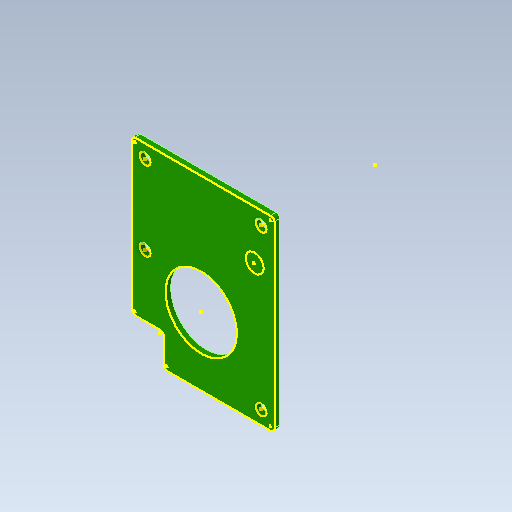
# Autodesk Inventor part: LED_PCB
Saved by Autodesk Inventor 2021 (Build 250183000, 183)
## iProperties
Created: 2020-02-27
Part Number: LED_PCB
Material: Generic
Document SubType Name: Modeling
Designer: lgnds
Density: 1 g/cm^3
Appearance: Default
Author: lgnds
Autodesk Inventor part; units mm, degrees
ref_plane "YZ Plane" through (0, 0, 0) normal (1, 0, 0) x (0, 1, 0)
ref_plane "XZ Plane" through (0, 0, 0) normal (0, 1, 0) x (-1, 0, 0)
ref_plane "XY Plane" through (0, 0, 0) normal (0, 0, 1) x (1, 0, 0)
sketch "Sketch1" plane through (0, 0, 0) normal (0, 0, 1) x (1, 0, 0)
  line L0 (-69, -79.6965) -> (69, -79.6965)
  line L1 (69, -79.6965) -> (69, 79.6965)
  line L2 (69, 79.6965) -> (-69, 79.6965)
  line L3 (-69, 79.6965) -> (-69, -79.6965)
  line L4 (-69, -79.6965) -> (69, 79.6965) construction
  line L5 (69, -79.6965) -> (-69, 79.6965) construction
  point P0 (0, 0)
  dimension "d0" = 138
  dimension "d1" = 159.393
  constraints: 12 end point, 2 midpoint, 2 parallel, 1 horizontal, 1 perpendicular
  measures "d0" distance of L1.end L2.end
  measures "d1" distance of L2.end L0.start
extrude "Extrusion1" add sketch "Sketch1" along normal blind 1.6
sketch "Sketch2" plane through (0, 0, 1.6) normal (0, 0, 1) x (1, 0, 0)
  line L0 (-69, -79.6965) -> (69, -79.6965) projected
  line L1 (69, -79.6965) -> (-23, -79.6965)
  line L2 (-23, -79.6965) -> (-23, -26.0895)
  line L3 (-23, -26.0895) -> (69, -26.0895)
  line L4 (69, -26.0895) -> (69, -79.6965)
  point P0 (0, 0)
  dimension "d4" = 53.607
  dimension "d5" = 92
  constraints: 8 end point, 2 parallel, 1 horizontal, 1 perpendicular
  measures "d4" distance between parallel lines of L3 L0
  measures "d5" distance of L2.end L3.end
extrude "Extrusion2" cut sketch "Sketch2" against normal blind 1.6
sketch "Sketch3" plane through (0, 0, 1.6) normal (0, 0, 1) x (1, 0, 0)
  line L0 (-86.2964, 75.1965) -> (76.951, 75.1965) construction
  line L1 (69, 79.6965) -> (-69, 79.6965) projected
  circle A0 centre (-42, 75.1965) radius 1.6
  circle A1 centre (42, 75.1965) radius 1.6
  line L2 (-69, 79.6965) -> (-69, -79.6965) projected
  line L3 (69, -26.0895) -> (69, 79.6965) projected
  point P0 (0, 0)
  dimension "d8" = 4.5
  dimension "d9" = 27
  dimension "d10" = 27
  dimension "d11" = 3.2
  dimension "d12" = 3.2
  constraints: 2 centre point, 2 end point, 2 point on line, 1 horizontal
  measures "d8" distance between parallel lines of L1 L0
  measures "d9" distance from line of L2 A0.centre
  measures "d10" distance from line of L3 A1.centre
  measures "d11" diameter of A0
  measures "d12" diameter of A1
extrude "Extrusion3" cut sketch "Sketch3" against normal blind 1.6
sketch "Sketch4" plane through (0, 0, 1.6) normal (0, 0, 1) x (1, 0, 0)
  circle A0 centre (-64.5, 12.6965) radius 2 construction
  circle A1 centre (-64.5, 62.6965) radius 2 construction
  circle A2 centre (0, 75.1965) radius 1.5 construction
  circle A3 centre (64.5, 52.6965) radius 1.5 construction
  circle A4 centre (64.5, 23) radius 1.5 construction
  circle A5 centre (64.5, -21.1966) radius 1.5 construction
  circle A6 centre (42, -21.1966) radius 1.5 construction
  circle A7 centre (0, -21.1966) radius 1.5 construction
  circle A8 centre (-32, -30.1966) radius 1.5 construction
  circle A9 centre (-32, -75.1966) radius 1.5 construction
  circle A10 centre (-64.5, -52.6966) radius 1.5 construction
  circle A11 centre (-64.5, -30.1966) radius 1.5 construction
  circle A12 centre (-64.5, 23) radius 1.5 construction
  circle A13 centre (-64.5, 52.6965) radius 1.5 construction
  circle A14 centre (-48.8035, -60) radius 7.75 construction
  arc A15 (-64.5, 57.6965) -> (-64.5, 67.6965) centre (-64.5, 62.6965) ccw
  line L0 (-64.5, 67.6965) -> (-69, 67.6965)
  line L1 (-64.5, 57.6965) -> (-69, 57.6965)
  line L2 (-69, 57.6965) -> (-69, 67.6965)
  line L3 (-69, 79.6965) -> (-69, -79.6965) projected
  line L4 (-105.8157, 37.6965) -> (-26.8283, 37.6965) construction
  circle A16 centre (-64.5, 52.6965) radius 1.6
  circle A17 centre (0, 75.1965) radius 1.6
  circle A18 centre (64.5, 52.6965) radius 1.6
  circle A19 centre (-64.5, 12.6965) radius 2 construction
  arc A20 (-64.5, 7.6965) -> (-64.5, 17.6965) centre (-64.5, 12.6965) ccw
  line L5 (-64.5, 7.6965) -> (-69, 7.6965)
  line L6 (-64.5, 17.6965) -> (-69, 17.6965)
  line L7 (-69, 17.6965) -> (-69, 7.6965)
  circle A21 centre (64.5, 23) radius 1.6
  circle A22 centre (64.5, -21.1966) radius 1.6
  circle A23 centre (42, -21.1966) radius 1.6
  circle A24 centre (0, -21.1966) radius 1.6
  circle A25 centre (-64.5, -52.6966) radius 1.6
  circle A26 centre (-32, -75.1966) radius 1.5
  circle A27 centre (-48.8035, -60) radius 10
  circle A28 centre (-64.5, 23) radius 1.6
  point P0 (0, 0)
  point P1 (-69, 62.6965)
  point P2 (-69, 12.6965)
  point P3 (-69, -4.3035)
  dimension "d15" = 10
  dimension "d16" = 25
  dimension "d17" = 50
  dimension "d18" = 3.2
  dimension "d19" = 3.2
  dimension "d20" = 3.2
  dimension "d23" = 3.2
  dimension "d24" = 3.2
  dimension "d25" = 3.2
  dimension "d26" = 3.2
  dimension "d27" = 3.2
  dimension "d28" = 20
  dimension "d29" = 3.2
  constraints: 14 centre point, 14 end point, 13 coincident, 8 symmetric about line, 4 point on circle, 3 horizontal, 2 tangent, 1 concentric, 1 midpoint, 1 point on line, 1 vertical, 2 other
  measures "d15" diameter of A15
  measures "d16" distance from line of L4 A1.centre
  measures "d17" distance of A1.centre A0.centre
  measures "d18" diameter of A16
  measures "d19" diameter of A17
  measures "d20" diameter of A18
  measures "d23" diameter of A24
  measures "d24" diameter of A23
  measures "d25" diameter of A22
  measures "d26" diameter of A21
  measures "d27" diameter of A25
  measures "d28" diameter of A27
  measures "d29" diameter of A28
extrude "Extrusion4" cut sketch "Sketch4" against normal up to next
sketch "Sketch5" plane through (0, 0, 1.6) normal (0, 0, 1) x (1, 0, 0)
  line L0 (-69, -79.6965) -> (-23, -79.6965) projected
  line L1 (-23, -26.0895) -> (-27.5, -26.0895)
  line L2 (-27.5, -26.0895) -> (-27.5, -79.6965)
  line L3 (-27.5, -79.6965) -> (-23, -79.6965)
  line L4 (-23, -79.6965) -> (-23, -26.0895)
  circle A0 centre (-32, -30.1966) radius 1.6 projected
  point P0 (0, 0)
  dimension "d32" = 4.5
  constraints: 8 end point, 2 parallel, 1 horizontal, 1 perpendicular, 1 point on line
  measures "d32" distance from line of L2 A0.centre
extrude "Extrusion5" cut sketch "Sketch5" against normal up to next contours L2 L1 L4 L0
thicken "Thicken1" operation add thickness 0.5 both sides no extend neighbours yes toward (0, 1, 0) faces at (-55.1667, -79.6965, 0.5333) (-69, -21.4345, 0.5333) (-27.5, -43.9585, 1.0667) (4.6667, -26.0895, 1.0667) (69, 9.1725, 0.5333) (23, 79.6965, 1.0667) (-69, 75.6965, 0.5333)
thicken "Thicken2" operation add thickness 0.5 both sides no extend neighbours yes toward (1, 0, 0) faces at (-69, 44.3632, 0.5333)
sketch "Sketch8" plane through (0, 0, 1.6) normal (0, 0, 1) x (1, 0, 0)
  line L0 (-28.25, -78.9465) -> (-28.25, -25.3395) projected
  line L1 (-68.25, -78.9465) -> (-28.25, -78.9465)
  line L2 (-28.25, -78.9465) -> (-28.25, -26.8395)
  line L3 (-28.25, -26.8395) -> (-68.25, -26.8395)
  line L4 (-68.25, -26.8395) -> (-68.25, -78.9465)
  line L5 (-28.25, -25.3395) -> (68.25, -25.3395) projected
  line L6 (-124.8564, 114.9316) -> (183.7235, 114.9316)
  line L7 (183.7235, 114.9316) -> (183.7235, -144.7335)
  line L8 (183.7235, -144.7335) -> (-124.8564, -144.7335)
  line L9 (-124.8564, -144.7335) -> (-124.8564, 114.9316)
  point P0 (0, 0)
  dimension "d47" = 1.5
  constraints: 16 end point, 4 parallel, 2 horizontal, 2 perpendicular, 1 point on line
  measures "d47" distance between parallel lines of L5 L3
extrude "Extrusion8" cut sketch "Sketch8" against normal blind 10
fillet "Fillet1" radius 1 3 edges at (-28.25, -78.9465, 0.8) (-28.25, -26.8395, 0.8) (-68.25, -26.8395, 0.8)
sketch "Sketch9" plane through (0, 0, 1.6) normal (0, 0, 1) x (1, 0, 0)
  line L0 (-68.25, -27.8395) -> (-68.25, -78.9465) projected
  line L1 (-68.25, -78.9465) -> (-59.25, -78.9465)
  line L2 (-59.25, -78.9465) -> (-59.25, -69.9465)
  line L3 (-59.25, -69.9465) -> (-68.25, -69.9465)
  line L4 (-68.25, -69.9465) -> (-68.25, -78.9465)
  point P0 (0, 0)
  dimension "d53" = 9
  dimension "d54" = 9
  constraints: 8 end point, 2 parallel, 1 horizontal, 1 perpendicular
  measures "d53" distance of L2.end L3.end
  measures "d54" distance of L1.end L2.end
extrude "Extrusion9" cut sketch "Sketch9" against normal blind 10
fillet "Fillet3" radius 1 3 edges at (-68.25, -69.9465, 0.8) (-59.25, -69.9465, 0.8) (-59.25, -78.9465, 0.8)
sketch "Sketch10" plane through (0, 0, 1.6) normal (0, 0, 1) x (1, 0, 0)
  circle A0 centre (-64.5, -30.5895) radius 1.6
  circle A1 centre (-32, -30.5895) radius 1.6
  circle A2 centre (-64.5, -52.6966) radius 1.6 projected
  line L0 (-68.25, -27.8395) -> (-68.25, -68.9465) projected
  line L1 (-29.25, -26.8395) -> (-67.25, -26.8395) projected
  line L2 (-28.25, -77.9465) -> (-28.25, -27.8395) projected
  point P0 (0, 0)
  dimension "d58" = 3.2
  dimension "d59" = 3.2
  dimension "d60" = 3.2
  dimension "d61" = 3.75
  dimension "d62" = 3.75
  dimension "d63" = 3.75
  dimension "d64" = 3.75
  dimension "d65" = 3.75
  constraints: 2 centre point
  measures "d58" diameter of A2
  measures "d59" diameter of A0
  measures "d60" diameter of A1
  measures "d61" distance from line of L0 A0.centre
  measures "d62" distance from line of L0 A2.centre
  measures "d63" distance from line of L1 A0.centre
  measures "d64" distance from line of L2 A1.centre
  measures "d65" distance from line of L1 A1.centre
extrude "Extrusion10" cut sketch "Sketch10" against normal up to next contours A0 | A1
sketch "OUTLINE" plane through (0, 0, 1.6) normal (0, 0, 1) x (1, 0, 0)
  line L0 (-29.25, -26.8395) -> (-67.25, -26.8395) projected
  arc A0 (-28.25, -27.8395) -> (-29.25, -26.8395) centre (-29.25, -27.8395) ccw projected
  line L1 (-28.25, -77.9465) -> (-28.25, -27.8395) projected
  arc A1 (-29.25, -78.9465) -> (-28.25, -77.9465) centre (-29.25, -77.9465) ccw projected
  line L2 (-58.25, -78.9465) -> (-29.25, -78.9465) projected
  arc A2 (-59.25, -77.9465) -> (-58.25, -78.9465) centre (-58.25, -77.9465) ccw projected
  line L3 (-59.25, -70.9465) -> (-59.25, -77.9465) projected
  arc A3 (-59.25, -70.9465) -> (-60.25, -69.9465) centre (-60.25, -70.9465) ccw projected
  line L4 (-67.25, -69.9465) -> (-60.25, -69.9465) projected
  arc A4 (-68.25, -68.9465) -> (-67.25, -69.9465) centre (-67.25, -68.9465) ccw projected
  line L5 (-68.25, -27.8395) -> (-68.25, -68.9465) projected
  arc A5 (-67.25, -26.8395) -> (-68.25, -27.8395) centre (-67.25, -27.8395) ccw projected
  circle A6 centre (-48.8035, -60) radius 10 projected
  point P0 (0, 0)
sketch "EXTRA" plane through (0, 0, 1.6) normal (0, 0, 1) x (1, 0, 0)
  circle A0 centre (-64.5, -30.5906) radius 1.5 projected
  circle A1 centre (-64.5, -52.6966) radius 1.5 projected
  circle A2 centre (-32, -75.1966) radius 1.5 projected
  circle A3 centre (-32, -30.5906) radius 1.5 projected
  circle A4 centre (-33.8026, -40.4918) radius 2.54 projected
  point P0 (0, 0)
equation "\"d10\" = d9"
equation "\"d12\" = d11"
equation "\"d16\" = 0.5 * d17"
equation "\"d19\" = d18"
equation "\"d20\" = d18"
equation "\"d23\" = d18"
equation "\"d24\" = d20"
equation "\"d25\" = d20"
equation "\"d26\" = d20"
equation "\"d27\" = d21"
equation "\"d29\" = d18"
equation "\"d54\" = d53"
equation "\"d59\" = d58"
equation "\"d60\" = d58"
equation "\"d61\" = d62"
equation "\"d63\" = d62"
equation "\"d64\" = d62"
equation "\"d65\" = d62"
equation "\"d21\" = d18"
body "Solid1"
